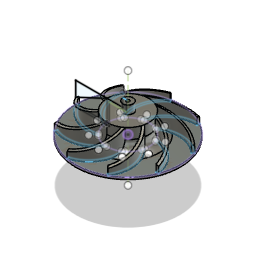
rotor v15 (Autodesk Fusion 360 design; units mm, degrees)
Autodesk Fusion 360 part; units mm, degrees
sketch "Sketch1" plane through (0, 0, 0) normal (0, 0, 1) x (1, 0, 0)
  line L0 (0, 45) -> (0, -50) construction
  line L1 (-1.5, 10) -> (-1.5, 20)
  line L2 (-1.5, 20) -> (-5, 20)
  line L3 (-5, 20) -> (-5, 12)
  line L4 (-5, 12) -> (-20, 12)
  line L5 (-20, 12) -> (-20, -8)
  line L6 (-20, -8) -> (-50, -8)
  line L7 (-50, -8) -> (-50, -10)
  line L8 (-50, -10) -> (-18, -10)
  line L9 (-18, -10) -> (-18, 10)
  line L10 (-18, 10) -> (-1.5, 10)
  line L11 (-20, 12) -> (-50, -2)
  line L12 (-50, -2) -> (-50, 12)
  line L13 (-50, 12) -> (-20, 12)
  dimension "d1" = 1.5
  dimension "d2" = 5
  dimension "d3" = 18
  dimension "d4" = 2
  dimension "d5" = 20
  dimension "d6" = 2
  dimension "d7" = 2
  dimension "d8" = 50
  dimension "d16" = 6
  constraint vertical L0
  constraint vertical L1
  constraint perpendicular L1 L2
  constraint perpendicular L2 L3
  constraint perpendicular L1 L4
  constraint perpendicular L4 L5
  constraint perpendicular L1 L6
  constraint perpendicular L6 L7
  constraint perpendicular L1 L8
  constraint perpendicular L6 L9
  constraint perpendicular L1 L10
  constraint perpendicular L6 L12
  constraint perpendicular L5 L13
  constraint collinear L7 L12
  measures "d1" distance of L0 L1
  measures "d2" distance of L0 L3
  measures "d3" distance of L0 L9
  measures "d4" distance of L5 L9
  measures "d5" distance of L8 L10
  measures "d6" distance of L6 L8
  measures "d7" distance of L4 L10
  measures "d8" distance of L0 L7
  measures "d16" distance of L6 L11.end
revolve "Revolve1" add sketch "Sketch1" angle 360 about axis through (0, 45, 0) along (0, -1, 0) contours L1 L2 L3 L4 L5 L6 L7 L8 L9 L10 makes body 1
fillet "Fillet2" radius 10 1 edges at (-18.6465, -8, 7.2323) on bodies 1
sketch "Sketch2" plane through (0, -8, 0) normal (0, 1, 0) x (-1, 0, 0)
  circle A0 centre (0, 0) radius 20
  circle A1 centre (0, 0) radius 50
  arc A2 (37.9867, -32.5117) -> (19.7355, 3.2417) centre (7.528, -25.525) ccw
  arc A3 (35.8376, -31.8602) -> (19.9887, 0.6724) centre (7.528, -25.525) ccw
  line L0 (37.9867, -32.5117) -> (35.8376, -31.8602)
  arc A4 (49.9976, -0.488) -> (13.0345, 15.1691) centre (22.1739, -14.7144) ccw
  arc A5 (47.9325, -1.3704) -> (14.88, 13.3635) centre (22.1739, -14.7144) ccw
  line L1 (49.9976, -0.488) -> (47.9325, -1.3704)
  arc A6 (38.6141, 31.764) -> (0.2345, 19.9986) centre (26.4444, 2.9812) ccw
  arc A7 (37.5993, 29.7607) -> (2.8089, 19.8018) centre (26.4444, 2.9812) ccw
  line L2 (38.6141, 31.764) -> (37.5993, 29.7607)
  arc A8 (9.1626, 49.1533) -> (-12.6752, 15.4706) centre (18.3413, 19.2819) ccw
  arc A9 (9.673, 46.9664) -> (-10.5766, 16.9745) centre (18.3413, 19.2819) ccw
  line L3 (9.1626, 49.1533) -> (9.673, 46.9664)
  arc A10 (-24.5761, 43.5432) -> (-19.6541, 3.7037) centre (1.6561, 26.5603) ccw
  arc A11 (-22.7795, 42.196) -> (-19.0132, 6.2047) centre (1.6561, 26.5603) ccw
  line L4 (-24.5761, 43.5432) -> (-22.7795, 42.196)
  arc A12 (-46.8155, 17.5588) -> (-17.4366, -9.7962) centre (-15.804, 21.4109) ccw
  arc A13 (-44.5732, 17.6816) -> (-18.5533, -7.4684) centre (-15.804, 21.4109) ccw
  line L5 (-46.8155, 17.5588) -> (-44.5732, 17.6816)
  arc A14 (-47.1493, -16.6416) -> (-7.0603, -18.7123) centre (-25.8693, 6.2431) ccw
  arc A15 (-45.5105, -15.1062) -> (-9.4121, -17.6469) centre (-25.8693, 6.2431) ccw
  line L6 (-47.1493, -16.6416) -> (-45.5105, -15.1062)
  arc A16 (-25.4215, -43.0552) -> (6.6195, -18.8728) centre (-23.83, -11.846) ccw
  arc A17 (-25.1531, -40.8256) -> (4.1331, -19.5683) centre (-23.83, -11.846) ccw
  line L7 (-25.4215, -43.0552) -> (-25.1531, -40.8256)
  arc A18 (8.2014, -49.3228) -> (17.202, -10.2024) centre (-10.6404, -24.3921) ccw
  arc A19 (6.9738, -47.4423) -> (15.7444, -12.3334) centre (-10.6404, -24.3921) ccw
  line L8 (8.2014, -49.3228) -> (6.9738, -47.4423)
  dimension "d29" = 360
  constraint coincident A1 A2.start
  constraint coincident A0 A2.end
  constraint concentric A2 A3
  constraint coincident A0 A3.end
extrude "Extrude1" add sketch "Sketch2" along normal up to surface (20 mm away) contours A0 A2 A3 L0 | A0 A18 A19 L8 | A0 A4 A5 L1 | A0 A16 A17 L7 | A0 A14 A15 L6 | A0 A6 A7 L2 | A0 A12 A13 L5 | A0 A10 A11 L4 | A0 A8 A9 L3 bodies 1
revolve "Revolve2" cut sketch "Sketch1" angle 360 about axis through (0, 45, 0) along (0, -1, 0) contours L11 L12 L13 bodies 1
fillet "Fillet1" radius 2 1 edges at (-16.7819, 10, 6.5091) on bodies 1
fillet "Fillet3" radius 12 1 edges at (-16.7819, -10, 6.5091) on bodies 1
copy_body "Body->Comp1" bodies 1 removing the originals makes body 2 in component "rotor"
component "rotor" placed x (1, 0, 0) y (0, 1, 0) z (0, 0, 1) at (0, 0, 0)
named bodies: "rotor"
